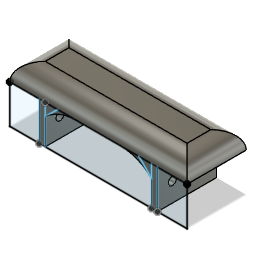
Aluminum Tower Cap v2 (Autodesk Fusion 360 design; units mm, degrees)
Autodesk Fusion 360 part; units mm, degrees
sketch "Sketch1" plane through (0, 0, 0) normal (0, 1, 0) x (1, 0, 0)
  line L0 (0, 0) -> (120, 0)
  line L1 (120, 0) -> (120, 40)
  line L2 (120, 40) -> (0, 40)
  line L3 (0, 40) -> (0, 0)
  dimension "d1" = 120
  dimension "d2" = 40
  constraint horizontal L0
  constraint vertical L1
  constraint horizontal L2
  constraint vertical L3
  constraint coincident L0.start L3.end
  measures "d1" distance of L1.end L2.end
  measures "d2" distance of L0.start L2.end
extrude "Extrude1" add sketch "Sketch1" along normal blind 38.1
fillet "Fillet1" radius 12 4 edges at (120, 38.1, -20) (60, 38.1, -40) (0, 38.1, -20) (60, 38.1, 0)
sketch "Sketch2" plane through (0, 0, 0) normal (0, 0, 1) x (1, 0, 0)
  line L0 (120, 26.1) -> (0, 26.1)
  line L1 (0, 26.1) -> (0, 0)
  line L2 (0, 0) -> (120, 0)
  line L3 (120, 0) -> (120, 26.1)
  line L4 (0, 26.1) -> (20, 26.1)
  line L5 (20, 26.1) -> (20, 0)
  line L6 (20, 0) -> (0, 0)
  line L7 (0, 0) -> (0, 26.1)
  line L8 (120, 26.1) -> (100, 26.1)
  line L9 (100, 26.1) -> (100, 0)
  line L10 (100, 0) -> (120, 0)
  line L11 (120, 0) -> (120, 26.1)
  line L12 (24, 26.1) -> (96, 26.1)
  line L13 (96, 26.1) -> (96, 0)
  line L14 (96, 0) -> (24, 0)
  line L15 (24, 0) -> (24, 26.1)
  line L16 (96, 17.5267) -> (87.4147, 26.1)
  line L17 (24, 17.6884) -> (32.4054, 26.1)
  dimension "d7" = 4
  dimension "d8" = 4
  constraint horizontal L4
  constraint vertical L5
  constraint horizontal L6
  constraint vertical L7
  constraint coincident L2 L5.end
  constraint coincident L0.end L1.start
  constraint horizontal L8
  constraint vertical L9
  constraint horizontal L10
  constraint vertical L11
  constraint coincident L2 L9.end
  constraint coincident L0.start L3.end
  constraint horizontal L12
  constraint vertical L13
  constraint horizontal L14
  constraint vertical L15
  constraint coincident L2 L13.end
  constraint coincident L0 L12.start
  constraint coincident L13 L16.start
  constraint coincident L12 L16.end
  constraint coincident L15 L17.start
  constraint coincident L12 L17.end
  measures "d7" distance of L5 L15
  measures "d8" distance of L9 L13
extrude "Extrude2" cut sketch "Sketch2" against normal blind 60 contours L0 L2 L3 L8 L9 L10 L11 | L0 L12 L13 L16 | L0 L2 L12 L13 L14 L15 L16 L17 | L0 L12 L15 L17 | L0 L1 L2 L4 L5 L6 L7
sketch "Sketch4" plane through (100, 0, 0) normal (1, 0, 0) x (0, 0, -1)
  line L0 (40, 0) -> (40, 26.1)
  line L1 (40, 26.1) -> (0, 26.1)
  line L2 (0, 26.1) -> (0, 0)
  line L3 (0, 0) -> (40, 0)
  line L4 (0, 13.05) -> (40, 13.05) construction
  circle A0 centre (10, 13.05) radius 2.75
  circle A1 centre (30, 13.05) radius 2.75
  line L5 (10, 13.05) -> (0, 13.05)
  line L6 (30, 13.05) -> (40, 13.05)
  dimension "d25" = 20
  dimension "d26" = 5.5
  dimension "d27" = 5.5
  constraint midpoint L2 L4.start
  constraint midpoint L0 L4.end
  constraint coincident L4 A0.centre
  constraint coincident L4 A1.centre
  constraint coincident A0.centre L5.start
  constraint parallel L4 L5
  constraint coincident A1.centre L6.start
  constraint perpendicular L0 L6
  constraint equal L5 L6
  measures "d25" distance of A0.centre A1.centre
  measures "d26" diameter of A0
  measures "d27" diameter of A1
extrude "Extrude3" cut sketch "Sketch4" against normal blind 97 contours A0 | A1
extrude "Extrude4" add sketch "Sketch2" against normal blind 40 contours L0 L12 L13 L16 | L0 L12 L15 L17
fillet "Fillet2" radius 30.5 2 edges at (32.4054, 26.1, -20) (87.4147, 26.1, -20)
